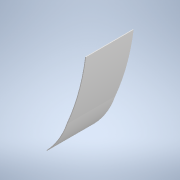
# Autodesk Inventor part: Bottom Lexan Ramp
Saved by Autodesk Inventor 2022 (Build 260153070, 153G)
## iProperties
Created: 2021-07-03
Part Number: Bottom Lexan Ramp
Material: Polycarbonate, Clear
Document SubType Name: Modeling
Designer: Main Account
Density: 1.2 g/cm^3
Appearance: Polycarbonate - Clear
Author: Main Account
Autodesk Inventor part; units mm, degrees
ref_plane "YZ Plane" through (0, 0, 0) normal (1, 0, 0) x (0, 1, 0)
ref_plane "XZ Plane" through (0, 0, 0) normal (0, 1, 0) x (-1, 0, 0)
ref_plane "XY Plane" through (0, 0, 0) normal (0, 0, 1) x (1, 0, 0)
sketch "Sketch1" plane through (0, 0, 0) normal (0, 0, 1) x (1, 0, 0)
  arc A0 (-16.5719, 1.6749) -> (27.0317, 73.4838) centre (-157.4047, 136.334) ccw
  arc A1 (27.0317, 73.4838) -> (66.2957, 215.9257) centre (-466.9704, 286.2877) ccw
  line L0 (-16.5719, 1.6749) -> (-18.1594, 1.6749)
  line L1 (66.2957, 215.9257) -> (64.7082, 215.9257)
  arc A2 (25.4442, 73.4838) -> (64.7082, 215.9257) centre (-468.558, 286.2877) ccw
  arc A3 (-18.1594, 1.6749) -> (25.4442, 73.4838) centre (-158.9922, 136.334) ccw
  dimension "d0" = 1.5875
  dimension "d2" = 1.5875
  dimension "d3" = 537.8882
  dimension "d4" = 194.851
  constraints: 8 point on circle, 4 centre point, 4 end point, 2 horizontal
  measures "d0" distance of L0.start L0.end
  measures "d2" distance of L1.start L1.end
  measures "d3" radius of A2
  measures "d4" radius of A3
extrude "Extrusion1" add sketch "Sketch1" against normal blind 101.6
body "Solid1"
